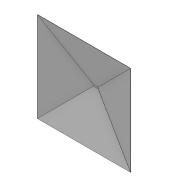
# Autodesk Inventor part: chimneyRoof
Saved by Autodesk Inventor 2017 (Build 210142000, 142)
## iProperties
Created: 2016-12-02
Part Number: chimneyRoof
Material: Generic
Document SubType Name: Sheet Metal
Designer: krosie
Density: 1 g/cm^3
Appearance: Default
Sheet Metal Rule: Default
Author: krosie
Autodesk Inventor part; units mm, degrees
ref_plane "YZ Plane" through (0, 0, 0) normal (1, 0, 0) x (0, 1, 0)
ref_plane "XZ Plane" through (0, 0, 0) normal (0, 1, 0) x (-1, 0, 0)
ref_plane "XY Plane" through (0, 0, 0) normal (0, 0, 1) x (1, 0, 0)
sketch "Sketch20" plane through (0, 0, 0) normal (1, 0, 0) x (0, 1, 0)
  line L0 (-1.0403, 3.8823) -> (-51.7638, 193.1852)
  line L1 (0, 0) -> (195.9808, 0) construction
  line L2 (-1.0403, -3.8823) -> (-51.7638, -193.1852)
  line L3 (0, 0) -> (200, 0) construction
  arc A0 (-1.0403, -3.8823) -> (-1.0403, 3.8823) centre (-15.5291, 0) ccw
  line L4 (-50.7979, 193.444) -> (-0.0743, 4.1411)
  arc A1 (-0.0743, -4.1411) -> (-0.0743, 4.1411) centre (-15.5291, 0) ccw
  line L5 (-0.0743, -4.1411) -> (-50.7979, -193.444)
  line L6 (-50.7979, 193.444) -> (-51.7638, 193.1852)
  line L7 (-50.7979, -193.444) -> (-51.7638, -193.1852)
  dimension "d97" = 90
  dimension "d81" = 200
  dimension "d82" = 105
  dimension "d83" = 200
  dimension "d84" = 105
  dimension "d85" = 15
  dimension "d86" = 1
  dimension "d87" = 90
  dimension "d88" = 90
  constraints: 16 end point, 4 point on circle, 2 centre point, 2 horizontal, 2 point on line, 2 tangent, 1 equal length, 3 other
  measures "d81" distance of L1.start L0.end
  measures "d82" angle of L1 L0
  measures "d83" distance of L1.start L2.end
  measures "d84" angle of L2 L3
  measures "d85" radius of A0
  measures "d86" distance between parallel lines of L0 L4
  measures "d87" angle of L7 L5
  measures "d88" angle of L6 L4
extrude "Extrusion7" add sketch "Sketch20" along normal blind 400
sketch "Sketch21" plane through (0, 0, 0) normal (0, 0, 1) x (1, 0, 0)
  line L0 (0, -51.7638) -> (0, -1.0403) projected
  line L1 (0, -51.7638) -> (196.1177, 0.7858)
  line L2 (0, -51.7638) -> (210, -51.7638) construction
  line L3 (400, -50.7979) -> (400, -51.7638) projected
  line L4 (400, -51.7638) -> (203.8823, 0.7858)
  line L5 (400, -51.7638) -> (610, -51.7638) construction
  arc A0 (203.8823, 0.7858) -> (196.1177, 0.7858) centre (200, -13.7031) ccw
  line L6 (400, -51.7638) -> (400, 8.2362)
  line L7 (400, -0.0743) -> (400, -50.7979) projected
  line L8 (400, -51.7638) -> (460, -51.7638) construction
  line L9 (0, -51.7638) -> (0, 8.2362)
  line L10 (400, 8.2362) -> (0, 8.2362)
  point P0 (0, 0)
  dimension "d92" = 15
  dimension "d94" = 165
  dimension "d95" = 15
  dimension "d96" = 60
  dimension "d97" = 90
  constraints: 16 end point, 4 horizontal, 2 point on circle, 2 tangent, 1 centre point, 1 collinear, 1 perpendicular, 1 point on line
  measures "d92" angle of L2 L1
  measures "d94" angle of L5 L4
  measures "d95" radius of A0
  measures "d96" distance of L3.end L6.end
  measures "d97" angle of L8 L6
extrude "Extrusion8" cut sketch "Sketch21" along normal through all both and the other way through all
sketch "Sketch22" plane through (210.6971, -1.0403, 3.8823) normal (0.2588, 0.9659, 0) x (0.6947, -0.1862, 0.6947)
  line L0 (272.4776, 0) -> (269.9731, -2.779) projected
  line L1 (0, 0) -> (272.4776, 0) projected
  ellipse E0 centre (37.5672, 41.6848) end of major axis (79.252, 81.9492) minor radius 15 (-5.3944, 5.5847) -> (0, 0) ccw projected
  line L2 (4.0481, 277.8986) -> (-5.3944, 5.5847) projected
  line L3 (1.184, 275.492) -> (4.0481, 277.8986) projected
  line L4 (-8.2585, 3.178) -> (1.184, 275.492) projected
  ellipse E1 centre (37.5672, 41.6848) end of major axis (-6.8966, -1.2639) minor radius 16 (-8.2585, 3.178) -> (-2.5045, -2.779) ccw projected
  line L5 (269.9731, -2.779) -> (-2.5045, -2.779) projected
  line L6 (4.0481, 277.8986) -> (-5.3944, 5.5847) projected
  line L7 (4.0481, 277.8986) -> (272.4776, 0)
  point P0 (-149.272, -138.788)
  constraints: 2 end point, 2 other
extrude "Extrusion9" add sketch "Sketch22" along normal blind 1 contours L1 E0 L2 L7
sketch "Sketch24" plane through (0, -51.7638, 193.1852) normal (-0.2588, 0.9659, 0) x (0.6947, 0.1862, -0.6947)
  line L0 (0, 0) -> (272.4776, 0) projected
  line L1 (2.5045, -2.779) -> (0, 0) projected
  line L2 (274.9821, -2.779) -> (2.5045, -2.779) projected
  ellipse E0 centre (234.9104, 41.6848) end of major axis (279.3742, -1.2639) minor radius 16 (274.9821, -2.779) -> (280.7361, 3.178) ccw projected
  line L3 (271.2936, 275.492) -> (280.7361, 3.178) projected
  line L4 (268.4295, 277.8986) -> (271.2936, 275.492) projected
  line L5 (277.872, 5.5847) -> (268.4295, 277.8986) projected
  ellipse E1 centre (234.9104, 41.6848) end of major axis (193.2256, 81.9492) minor radius 15 (272.4776, 0) -> (277.872, 5.5847) ccw projected
  line L6 (277.872, 5.5847) -> (268.4295, 277.8986) projected
  line L7 (268.4295, 277.8986) -> (0, 0)
  point P0 (143.8509, 129.6415)
  constraints: 2 end point, 2 other
extrude "Extrusion10" add sketch "Sketch24" along normal blind 1 contours L7 L5 E1 L0
equation "\"BendRadius\" = Thickness"
equation "\"BendReliefWidth\" = Thickness"
equation "\"BendReliefDepth\" = 0.5 * Thickness"
equation "\"CornerReliefSize\" = 4 * Thickness"
equation "\"MinimumRemnant\" = 2 * Thickness"
equation "\"TransitionRadius\" = BendRadius"
equation "\"JacobiRadiusSize\" = Thickness"
equation "\"GapSize\" = Thickness"
equation "\"Thickness\" = 0.5"
body "Solid4"
